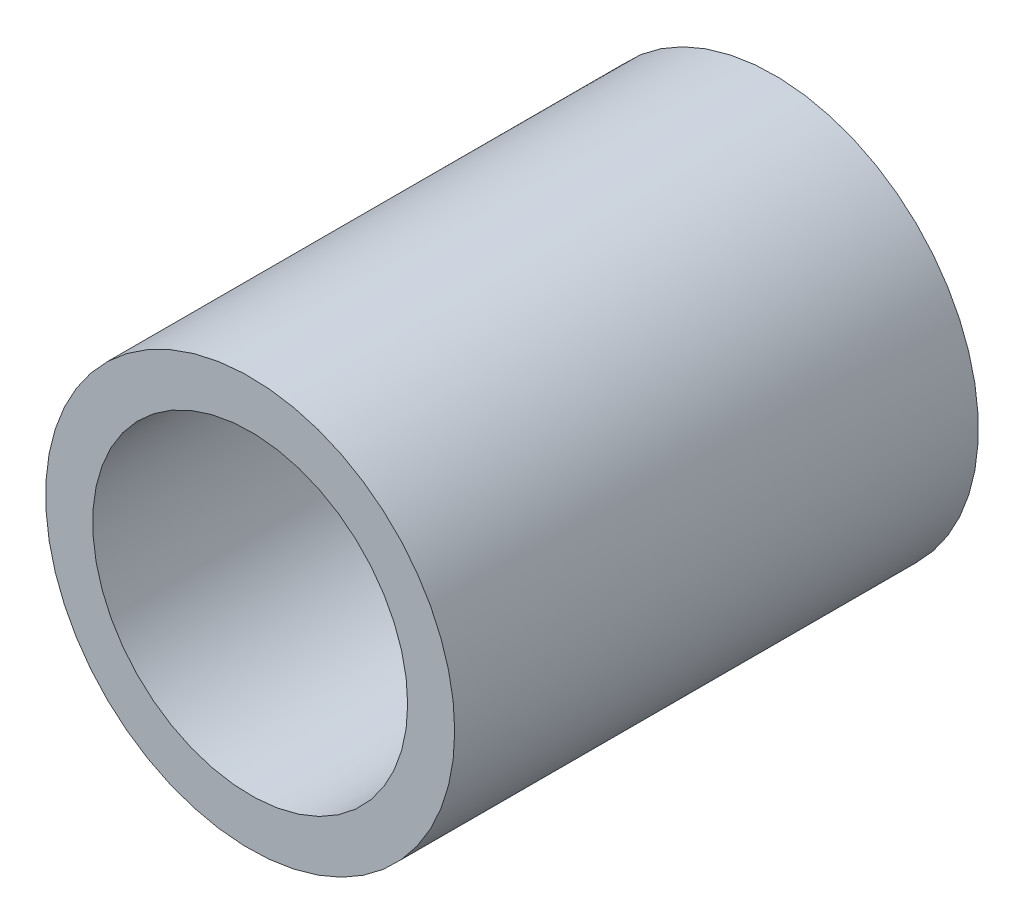
# Autodesk Inventor part: KB33-046-003-001 - Крепление
Saved by Autodesk Inventor 2019 (Build 230136000, 136)
## iProperties
Created: 2021-06-09
Part Number: KB33-046-003-001 - Крепление
Material: Типовые
Document SubType Name: Modeling
Designer: Петров Иван
Density: 1 g/cm^3
Appearance: По умолчанию
Author: Петров Иван
Autodesk Inventor part; units mm, degrees
ref_plane "YZ Plane" through (0, 0, 0) normal (1, 0, 0) x (0, 1, 0)
ref_plane "XZ Plane" through (0, 0, 0) normal (0, 1, 0) x (-1, 0, 0)
ref_plane "XY Plane" through (0, 0, 0) normal (0, 0, 1) x (1, 0, 0)
sketch "Sketch1" plane through (0, 0, 0) normal (0, 0, 1) x (1, 0, 0)
  circle A0 centre (0, 0) radius 19.25
  circle A1 centre (0, 0) radius 25
  dimension "d0" = 38.5
  dimension "d1" = 50
  constraints: 2 centre point, 2 coincident
  measures "d0" diameter of A0
  measures "d1" diameter of A1
extrude "Extrusion1" add sketch "Sketch1" along normal blind 60
sketch "Sketch2" plane through (0, 0, 0) normal (0, 0, -1) x (-1, 0, 0)
  circle A0 centre (0, 0) radius 25
  arc A1 (-9.9286, -5.8029) -> (-9.9286, 5.8029) centre (0, 0) ccw
  arc A2 (-9.9286, 5.8029) -> (-9.9286, -5.8029) centre (-7, 0) ccw
  circle A3 centre (0, -15) radius 1.25
  circle A4 centre (12.9904, -7.5) radius 1.25
  circle A5 centre (12.9904, 7.5) radius 1.25
  circle A6 centre (0, 15) radius 1.25
  circle A7 centre (-12.9904, 7.5) radius 1.25
  circle A8 centre (-12.9904, -7.5) radius 1.25
  circle A9 centre (-7, 0) radius 6
  arc A10 (-10.375, -4.9608) -> (-10.375, 4.9608) centre (-7, 0) ccw
  spline S0 degree 3 poles (-10.375, 4.9608) (-10.4487, 4.9106) (-10.5225, 4.858) (-10.5964, 4.8027) knots 0 0 0 0 1 1 1 1
  arc A11 (-10.5964, 4.8027) -> (-10.5964, -4.8027) centre (-7, 0) ccw
  spline S1 degree 3 poles (-10.5964, -4.8027) (-10.5225, -4.858) (-10.4487, -4.9106) (-10.375, -4.9608) knots 0 0 0 0 1 1 1 1
  dimension "d4" = 50
  constraints: 12 centre point, 8 point on circle, 37 other
  measures "d4" diameter of A0
extrude "Extrusion2" add sketch "Sketch2" along normal blind 4 contours A0 | A2 A1
sketch "Sketch3" plane through (0, 0, -4) normal (0, 0, -1) x (-1, 0, 0)
  arc A0 (-10.375, -4.9608) -> (-10.375, 4.9608) centre (-7, 0) ccw projected
  circle A1 centre (-7, 0) radius 6.5
  point P0 (0, 0)
  dimension "d7" = 13
  constraints: 1 centre point, 1 coincident
  measures "d7" diameter of A1
extrude "Extrusion3" cut sketch "Sketch3" against normal blind 4
body "Solid1"
